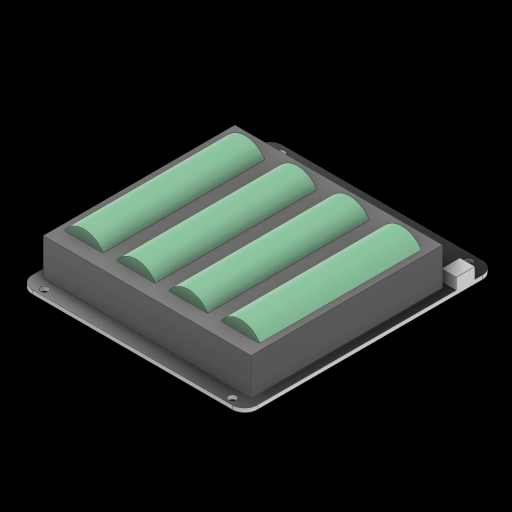
# Autodesk Inventor part: 010_Battery_2Cell
Saved by Autodesk Inventor 2024 (Build 280153000, 153)
## iProperties
Created: 2023-07-20
Part Number: 010_Battery_2Cell
Material: Generisch
Document SubType Name: Modeling
Designer: Philipp
Density: 1 g/cm^3
Appearance: Vorgabe
Author: Philipp
Autodesk Inventor part; units mm, degrees
ref_plane "YZ Plane" through (0, 0, 0) normal (1, 0, 0) x (0, 1, 0)
ref_plane "XZ Plane" through (0, 0, 0) normal (0, 1, 0) x (-1, 0, 0)
sketch "Skizze1" plane through (0, 0, 0) normal (0, 0, 1) x (1, 0, 0)
  line L0 (45.25, 50.25) -> (-45.25, 50.25)
  line L1 (-45.25, 50.25) -> (-45.25, -50.25)
  line L2 (-45.25, -50.25) -> (45.25, -50.25)
  line L3 (45.25, -50.25) -> (45.25, 50.25)
  line L4 (45.25, 50.25) -> (-45.25, -50.25) construction
  line L5 (-45.25, 50.25) -> (45.25, -50.25) construction
  point P0 (0, 0)
  dimension "d0" = 90.5
  dimension "d1" = 100.5
  constraints: 12 end point, 2 midpoint, 2 parallel, 1 horizontal, 1 perpendicular
  measures "d0" distance of L2.end L1.end
  measures "d1" distance of L1.end L0.end
extrude "Extrusion1" add sketch "Skizze1" along normal blind 1.6
fillet "Rundung1" radius 5 4 edges at (45.25, 50.25, 0.8) (-45.25, 50.25, 0.8) (45.25, -50.25, 0.8) (-45.25, -50.25, 0.8)
sketch "Skizze2" plane through (0, 0, 0) normal (0, 0, -1) x (-1, 0, 0)
  line L0 (-5.75, -11.25) -> (0.75, -11.25)
  line L1 (0.75, -11.25) -> (0.75, -17.75)
  line L2 (0.75, -17.75) -> (-5.75, -17.75)
  line L3 (-5.75, -17.75) -> (-5.75, -11.25)
  line L4 (-5.75, -11.25) -> (0.75, -17.75) construction
  line L5 (0.75, -11.25) -> (-5.75, -17.75) construction
  line L6 (40.25, -50.25) -> (-40.25, -50.25) projected
  line L7 (-45.25, -45.25) -> (-45.25, 45.25) projected
  point P0 (0, 0)
  point P1 (-2.5, -14.5)
  point P2 (-2.5, -17.75)
  dimension "d5" = 32.5
  dimension "d6" = 39.5
  dimension "d7" = 6.5
  dimension "d8" = 6.5
  constraints: 12 end point, 3 midpoint, 2 parallel, 1 horizontal, 1 perpendicular
  measures "d5" distance from line of L6 point (-2.5, -17.75)
  measures "d6" distance between parallel lines of L7 L3
  measures "d7" distance of L2.end L0.start
  measures "d8" distance of L0.start L0.end
extrude "Extrusion2" add sketch "Skizze2" along normal blind 5
fillet "Rundung2" radius 0.5 4 edges at (-0.75, -11.25, -2.5) (-0.75, -17.75, -2.5) (5.75, -17.75, -2.5) (5.75, -11.25, -2.5)
sketch "Skizze3" plane through (0, 0, 0) normal (0, 0, -1) x (-1, 0, 0)
  line L0 (38.25, -33.75) -> (45.25, -33.75)
  line L1 (45.25, -33.75) -> (45.25, -42.75)
  line L2 (45.25, -42.75) -> (38.25, -42.75)
  line L3 (38.25, -42.75) -> (38.25, -33.75)
  line L4 (38.25, -33.75) -> (45.25, -42.75) construction
  line L5 (45.25, -33.75) -> (38.25, -42.75) construction
  line L6 (40.25, -50.25) -> (-40.25, -50.25) projected
  line L7 (45.25, 45.25) -> (45.25, -45.25) projected
  point P0 (0, 0)
  point P1 (41.75, -38.25)
  dimension "d12" = 7.5
  dimension "d13" = 7
  dimension "d14" = 9
  constraints: 12 end point, 2 midpoint, 2 parallel, 1 collinear, 1 horizontal, 1 perpendicular
  measures "d12" distance between parallel lines of L6 L2
  measures "d13" distance of L1.end L2.end
  measures "d14" distance of L2.end L0.start
extrude "Extrusion3" add sketch "Skizze3" along normal blind 5
fillet "Rundung3" radius 2 2 edges at (-41.75, -33.75, -5) (-41.75, -42.75, -5)
sketch "Skizze4" plane through (0, 0, 1.6) normal (0, 0, 1) x (1, 0, 0)
  line L0 (39.25, 42.25) -> (45.25, 42.25)
  line L1 (45.25, 42.25) -> (45.25, 34.75)
  line L2 (45.25, 34.75) -> (39.25, 34.75)
  line L3 (39.25, 34.75) -> (39.25, 42.25)
  line L4 (39.25, 42.25) -> (45.25, 34.75) construction
  line L5 (45.25, 42.25) -> (39.25, 34.75) construction
  line L6 (45.25, -45.25) -> (45.25, 45.25) projected
  line L7 (-45.25, 45.25) -> (-45.25, -45.25) projected
  line L8 (40.25, 50.25) -> (-40.25, 50.25) projected
  line L9 (-43.25, 42.25) -> (-38.75, 42.25)
  line L10 (-38.75, 42.25) -> (-38.75, 33.25)
  line L11 (-38.75, 33.25) -> (-43.25, 33.25)
  line L12 (-43.25, 33.25) -> (-43.25, 42.25)
  line L13 (-43.25, 42.25) -> (-38.75, 33.25) construction
  line L14 (-38.75, 42.25) -> (-43.25, 33.25) construction
  point P0 (0, 0)
  point P1 (42.25, 38.5)
  point P2 (42.25, 42.25)
  point P3 (-41, 37.75)
  dimension "d19" = 8
  dimension "d20" = 7.5
  dimension "d21" = 6
  dimension "d22" = 8
  dimension "d23" = 9
  dimension "d24" = 4.5
  dimension "d25" = 2
  constraints: 24 end point, 5 midpoint, 4 parallel, 2 horizontal, 2 perpendicular, 1 collinear
  measures "d19" distance from line of L8 point (42.25, 42.25)
  measures "d20" distance of L2.end L0.start
  measures "d21" distance of L1.end L2.end
  measures "d22" distance between parallel lines of L8 L9
  measures "d23" distance of L9.end L10.end
  measures "d24" distance of L10.end L11.end
  measures "d25" distance between parallel lines of L7 L12
extrude "Extrusion4" add sketch "Skizze4" along normal blind 4.5
sketch "Skizze5" plane through (-43.25, 33.25, 1.6) normal (-1, 0, 0) x (0, 0, 1)
  line L0 (1.5, 1.5) -> (3.5, 1.5)
  line L1 (3.5, 1.5) -> (3.5, 7.5)
  line L2 (3.5, 7.5) -> (1.5, 7.5)
  line L3 (1.5, 7.5) -> (1.5, 1.5)
  line L4 (1.5, 1.5) -> (3.5, 7.5) construction
  line L5 (3.5, 1.5) -> (1.5, 7.5) construction
  line L6 (0, 9) -> (4.5, 9) projected
  line L7 (4.5, 9) -> (4.5, 0) projected
  point P0 (-1.6, -33.25)
  point P1 (2.5, 4.5)
  dimension "d28" = 1.5
  dimension "d29" = 6
  dimension "d30" = 1
  dimension "d31" = 2
  constraints: 12 end point, 2 midpoint, 2 parallel, 1 horizontal, 1 perpendicular
  measures "d28" distance between parallel lines of L6 L2
  measures "d29" distance of L0.end L1.end
  measures "d30" distance between parallel lines of L7 L1
  measures "d31" distance of L1.end L2.end
extrude "Extrusion5" add sketch "Skizze5" along normal blind 3
sketch "Skizze6" plane through (0, 0, 1.6) normal (0, 0, 1) x (1, 0, 0)
  line L0 (-41.75, 32.75) -> (41.75, 32.75)
  line L1 (41.75, 32.75) -> (41.75, -44.25)
  line L2 (41.75, -44.25) -> (-41.75, -44.25)
  line L3 (-41.75, -44.25) -> (-41.75, 32.75)
  line L4 (-41.75, 32.75) -> (41.75, -44.25) construction
  line L5 (41.75, 32.75) -> (-41.75, -44.25) construction
  line L6 (-40.25, -50.25) -> (40.25, -50.25) projected
  line L7 (-45.25, 45.25) -> (-45.25, -45.25) projected
  line L8 (45.25, -45.25) -> (45.25, 34.75) projected
  point P0 (0, 0)
  point P1 (0, -5.75)
  dimension "d34" = 6
  dimension "d35" = 3.5
  dimension "d36" = 3.5
  dimension "d37" = 77
  constraints: 12 end point, 2 midpoint, 2 parallel, 1 horizontal, 1 perpendicular
  measures "d34" distance between parallel lines of L6 L2
  measures "d35" distance between parallel lines of L7 L3
  measures "d36" distance between parallel lines of L8 L1
  measures "d37" distance of L0.end L1.end
extrude "Extrusion6" add sketch "Skizze6" along normal blind 15
ref_plane "Arbeitsebene1" through (-41.75, -38.25, 1.6) normal (0, -1, 0) x (1, 0, 0)
sketch "Skizze7" plane through (-41.75, -38.25, 1.6) normal (0, -1, 0) x (1, 0, 0)
  circle A0 centre (10.25, 10.4) radius 9
  circle A1 centre (31.25, 10.4) radius 9
  circle A2 centre (52.25, 10.4) radius 9
  circle A3 centre (73.25, 10.4) radius 9
  line L0 (1.5, -1.6) -> (82, -1.6) projected
  line L1 (10.25, 10.4) -> (114.75, 10.4) construction
  line L2 (0, 0) -> (83.5, 0) construction
  point P0 (41.75, -1.6)
  point P1 (62.5, 10.4)
  point P2 (41.75, 0)
  dimension "d41" = 18
  dimension "d42" = 18
  dimension "d43" = 18
  dimension "d44" = 18
  dimension "d45" = 21
  dimension "d46" = 21
  dimension "d47" = 21
  dimension "d49" = 31.5
  dimension "d50" = 21
  constraints: 4 centre point, 3 point on line, 2 end point, 2 midpoint, 1 horizontal
  measures "d41" diameter of A0
  measures "d42" diameter of A1
  measures "d43" diameter of A2
  measures "d44" diameter of A3
  measures "d46" distance of A1.centre L1.start
  measures "d47" distance of A2.centre A1.centre
  measures "d49" horizontal distance of point (41.75, 0) L1.start
  measures "d50" distance of A2.centre A3.centre
extrude "Extrusion7" add sketch "Skizze7" against normal blind 65
sketch "Skizze8" plane through (0, 0, 1.6) normal (0, 0, 1) x (1, 0, 0)
  line L0 (-37.75, 47.25) -> (37.75, 47.25)
  line L1 (37.75, 47.25) -> (37.75, -47.75)
  line L2 (37.75, -47.75) -> (-37.75, -47.75)
  line L3 (-37.75, -47.75) -> (-37.75, 47.25)
  line L4 (41.75, 32.75) -> (-41.75, 32.75) projected
  line L5 (40.25, 50.25) -> (-40.25, 50.25) projected
  point P0 (0, 0)
  point P1 (0, 32.75)
  point P2 (0, 47.25)
  dimension "d53" = 95
  dimension "d54" = 75.5
  dimension "d55" = 0
  dimension "d56" = 3
  constraints: 8 end point, 4 coincident, 2 midpoint, 2 parallel, 1 horizontal, 1 perpendicular
  measures "d53" distance of L2.end L0.start
  measures "d54" distance of L0.start L0.end
  measures "d55" horizontal distance of point (0, 32.75) point (0, 47.25)
  measures "d56" distance between parallel lines of L5 L0
hole "Bohrung1" at (-37.75, 47.25, 1.6) at (37.75, 47.25, 1.6) at (-37.75, -47.75, 1.6) at (37.75, -47.75, 1.6) direction (0, 0, -1) diameter 3 depth 1.6
equation "\"d49\" = 1.5 * d46"
